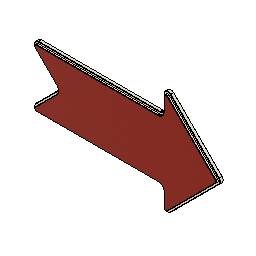
Arrows v4 (Autodesk Fusion 360 design; units mm, degrees)
Autodesk Fusion 360 part; units mm, degrees
sketch "Náčrt1" plane through (0, 0, 0) normal (0, 0, 1) x (1, 0, 0)
  line L0 (0, 0) -> (-50, 0) construction
  line L1 (0, 0) -> (-15, 15)
  line L2 (-15, 15) -> (-15, 8)
  line L3 (-15, 8) -> (-50, 8)
  line L4 (-15, -8) -> (-50, -8)
  line L5 (-15, -15) -> (-15, -8)
  line L6 (0, 0) -> (-15, -15)
  line L7 (-50, 8) -> (-42, 0)
  line L8 (-50, -8) -> (-42, 0)
  dimension "d1" = 50
  dimension "d2" = 35
  dimension "d4" = 15
  dimension "d5" = 8
  constraint coincident L0.start L1.start
  constraint horizontal L0
  constraint perpendicular L0 L2
  constraint perpendicular L2 L3
  constraint symmetric L0 L1.start L6.start
  constraint symmetric L0 L1.end L5.start
  constraint symmetric L0 L2.end L4.start
  constraint symmetric L0 L3.end L4.end
  constraint coincident L0 L7.end
  constraint parallel L1 L7
  constraint vertical L0.end L3.end
  measures "d1" distance of L0.start L0.end
  measures "d2" distance of L2.end L3.end
  measures "d4" vertical distance of L0.start L1.end
  measures "d5" distance of L0.end L7.end
extrude "Vysunutí1" add sketch "Náčrt1" along normal blind 1.4
fillet "Zaoblení1" radius 1 8 edges at (-50, 8, 0.7) (-50, -8, 0.7) (-15, -8, 0.7) (-15, -15, 0.7) (0, 0, 0.7) (-15, 15, 0.7) (-15, 8, 0.7) (-42, 0, 0.7)
ref_plane "PracovníRovina1" through (-30, 0, 0) normal (1, 0, 0) x (0, 1, 0)
sketch "Náčrt2" plane through (-30, 0, 0) normal (1, 0, 0) x (0, 0, -1)
  line L0 (-1.4, -8) -> (-1.4, -6.2929)
  line L1 (0, -8) -> (-1.4, -8)
  line L2 (-0.9, -8.5) -> (-1.9, -8.5)
  line L3 (-1.9, -8.5) -> (-1.9, -7.5)
  line L4 (-1.9, -7.5) -> (-0.9, -7.5)
  line L5 (-0.9, -7.5) -> (-0.9, -8.5)
  line L6 (-0.9, -8.5) -> (-1.9, -7.5) construction
  line L7 (-1.9, -8.5) -> (-0.9, -7.5) construction
  point P0 (-1.4, -8)
  point P1 (-1.4, -8)
  dimension "d13" = 1
  dimension "d14" = 1
  constraint horizontal L2
  constraint perpendicular L2 L3
  constraint parallel L2 L4
  constraint parallel L3 L5
  constraint coincident L6 P1
  constraint coincident L7 P1
  constraint coincident P1 P0
  measures "d13" distance of L3.end L4.end
  measures "d14" distance of L2.end L3.end
sweep "Tažení1" cut profiles "Náčrt2" along 16 edges at (-15.2929, -8.2929, 1.4) (-15, -10.7929, 1.4) (-14.3827, -13.5097, 1.4) (-7, -7, 1.4) (-0.4142, 0, 1.4) (-7, 7, 1.4) (-14.3827, 13.5097, 1.4) (-15, 10.7929, 1.4) (-15.2929, 8.2929, 1.4) (-31.7929, 8, 1.4) (-48.5097, 7.3827, 1.4) (-45.5, 3.5, 1.4) (-42.4142, 0, 1.4) (-45.5, -3.5, 1.4) (-48.5097, -7.3827, 1.4) (-31.7929, -8, 1.4) section 1 contours L0 L1 L4 L5
chamfer "Zkosení1" distance 0.1 angle 45 32 edges at (-31.7929, -7.5, 1.4) (-14.9393, -7.9393, 1.4) (-14.5, -10.7929, 1.4) (-14.1913, -13.0477, 1.4) (-7.3536, -6.6464, 1.4) (-0.9142, 0, 1.4) (-7.3536, 6.6464, 1.4) (-14.1913, 13.0477, 1.4) (-14.5, 10.7929, 1.4) (-14.9393, 7.9393, 1.4) (-31.7929, 7.5, 1.4) (-48.0477, 7.1913, 1.4) (-45.1464, 3.8536, 1.4) (-41.9142, 0, 1.4) (-45.1464, -3.8536, 1.4) (-48.0477, -7.1913, 1.4) (-31.7929, -8, 0.9) (-48.5097, -7.3827, 0.9) (-45.5, -3.5, 0.9) (-42.4142, 0, 0.9) (-45.5, 3.5, 0.9) (-48.5097, 7.3827, 0.9) (-31.7929, 8, 0.9) (-15.2929, 8.2929, 0.9) (-15, 10.7929, 0.9) (-14.3827, 13.5097, 0.9) (-7, 7, 0.9) (-0.4142, 0, 0.9) (-7, -7, 0.9) (-14.3827, -13.5097, 0.9) (-15, -10.7929, 0.9) (-15.2929, -8.2929, 0.9)
chamfer "Zkosení1" distance 0.1 angle 45 16 edges at (-31.7929, -8, 0) (-48.5097, -7.3827, 0) (-45.5, -3.5, 0) (-42.4142, 0, 0) (-45.5, 3.5, 0) (-48.5097, 7.3827, 0) (-31.7929, 8, 0) (-15.2929, 8.2929, 0) (-15, 10.7929, 0) (-14.3827, 13.5097, 0) (-7, 7, 0) (-0.4142, 0, 0) (-7, -7, 0) (-14.3827, -13.5097, 0) (-15, -10.7929, 0) (-15.2929, -8.2929, 0)
named bodies: "Arrow"
